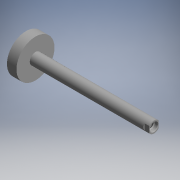
# Autodesk Inventor part: 536288 ADN-100-P-I_(KS)
Saved by Autodesk Inventor 2017.3 (Build 213256000, 256)
## iProperties
Part Number: 536288 ADN-100-P-I_(KS)
Material: Generic
Catalog Web Link: www.cadenas.de
Description: ADN-(KS)-Compact cylinder - piston rod
Vendor: FESTO
Document SubType Name: Modeling
Designer: partserver
Manufacturer: FESTO
Mass: 25.8333 g
Surface Area: 88.9082 cm^2
Volume: 25.8333 cm^3
Density: 1 g/cm^3
Appearance: PSOLRGB-191-191-191
Category: PARTsolutions
Company: FESTO
Title: 536288 ADN-100-P-I_(KS)
Author: Cadenas PARTsolutions
Comments: Compact cylinder - piston rod
PSOL_IDENT_0: {$CADENAS_DATA\23d-libs\festo\parts\a\adn\parts\adn_ks.prj},238 {VTYP=3D},{NB=536288 ADN-100-P-I_(KS
PSOL_IDENT_1: )},{LINA=536288 ADN-100-P-I_(KS)},{NN=ADN-(KS)},{DATE=20.11.2019 12:35:12},{GEOMDATE=08.01.2019 14:3
PSOL_IDENT_2: 4:57},{VERSION=},{LINEID=8210},{WBVAR=DF,HUB,TH,Q,S2S20,K2,K5,K8,K10,S1,TT,R8},{WBNUMERIC=HUB,K2,K8}
PSOL_IDENT_3: {NB=536288 ADN-100-P-I_(KS)},{LINA=536288 ADN-100-P-I_(KS)},{KT=536288},{TNR=536288},{AUSF=ADN},{D
PSOL_IDENT_4: F=P},{GA=A},{WHX=6.1},{WH0=6.100},{WH1=18.000},{WH2=12.500},{WH3=6.600},{WHX1=6.1},{WHX2=6.8},{WH=6.
PSOL_IDENT_5: 1},{ZM=58.600},{ZM2=59.700},{ZB=51.100},{ZB1=62.900},{ZB2=51.700},{ZB6=57.500},{ZA=45.000},{KDM=40},
PSOL_IDENT_6: {HUBP=-},{HUB=100},{HUB1=[1-400]},{HUB2=[1-300]},{HUB3=[10-400]},{HUB4=[1-400]},{TH=I},{THC='A','I'}
PSOL_IDENT_7: ,{Q=-},{VAR1C='-','Q'},{S2S20=-},{VAR2C='-','S2','S20'},{VAR22C='-','S2'},{VAR222C='-','S2'},{K2=0},
PSOL_IDENT_8: {VAR3C=0,[1-20]},{VAR33C=0},{K5=-},{K5A='-','M10','M12'},{K5I='-','M6'},{K5S1A='-','M10X1,25','M12'}
PSOL_IDENT_9: ,{K5S1I='-','M8'},{K5C='-','M6'},{K5N=0},{K5P=0},{K5T=},{K8=0},{K10=-},{K10A='-','K10'},{K10N=},{S1=
PSOL_IDENT_10: -},{TT=-},{TT1='-','TT'},{R8=-},{R81='-','R8'},{VAR4C=0,[1-400]},{VAR5C='-','S6'},{VAR6C='-','S1'},{
PSOL_IDENT_11: VAR66C='-','S1'},{VAR7C='-','R3'},{HUBALG=[1-400]},{A=19.000},{A1=22.000},{AF=16.000},{AF1=0.000},{A
PSOL_IDENT_12: F2=14.000},{AF3=20.000},{AF5=14.000},{AF7=16.000},{D8=4.500},{D9=8.000},{KF=M8},{KFN=8.000},{KF1=M10
PSOL_IDENT_13: },{KF1C=10.0000},{KF2=-},{KF2C=0.0000},{KF3=M6},{KF3C=6.0000},{KF5=M6},{KF5N=6},{KF7=M8},{KF7N=8},{K
PSOL_IDENT_14: K=M10X1.25},{KKN=10},{KKP=1.25},{KK1=M12X1.25},{KK1N=12.0000},{KK1P=1.25},{L2=45.000},{L8=3.000},{MM=
PSOL_IDENT_15: 12.000},{MM1=16.000},{PL=8.200},{SF=10},{SF1=13},{SF3=10.0},{WL=4.700},{WL1=6.500},{QN=},{S2N=},{S1N=
PSOL_IDENT_16: },{K2N=},{K8N=},{KKC3=8.200},{KKF2=0.600},{KKD5=1.500},{KKE2=20.000},{K5C3=0},{K5F2=0},{K5D5=0},{KK1
PSOL_IDENT_17: C3=10.200},{KK1F2=0.600},{KK1D5=1.500},{KK1E2=20.000},{L100S1=1.000},{L101S1=4.700},{L102S1=20.000},
PSOL_IDENT_18: {L103S1=24.000},{D100S1=10.500},{L100=0.400},{L101=3.300},{L102=16.000},{L103=20.000},{D100=8.400},{
PSOL_IDENT_19: L100Q=0.400},{L101Q=2.600},{L101K5=2.600},{L102Q=14.000},{L103Q=18.000},{D100Q=6.400},{L100S1K5=0.60
PSOL_IDENT_20: 0},{L101S1K5=3.300},{L102S1K5=16.000},{L103S1K5=21.000},{D100S1K5=8.400},{VERS=2},{TTN=},{R8N=},{D20=
PSOL_IDENT_21: 0.000},{XF31=4.000},{B31=5.000},{DFALG='P','PPS'}
NB: 536288 ADN-100-P-I_(KS)
NN: ADN-(KS)
NT: Compact cylinder - piston rod
NBSYN: $TNR. $AUSF.-$HUB.-$DF.-$TH.$QN.$S2N.$K2N.$K5T.$K8N.$K10N.$S1N.$TTN.$R8N._(KS)
LINA: 536288 ADN-100-P-I_(KS)
CATALOG: Festo
TNR: 536288
AUSF: ADN
DF: P
GA: A
WHX: 6.1
WH0: 6.1
WH1: 18
WH2: 12.5
WH3: 6.6
WHX1: 6.1
WHX2: 6.8
WH: 6.1
ZM: 58.6
ZM2: 59.7
ZB: 51.1
ZB1: 62.9
ZB2: 51.7
ZB6: 57.5
ZA: 45
KDM: 40
HUBP: -
HUB: 100
TH: I
Q: -
S2S20: -
K2: 0
K5: -
K8: 0
K10: -
S1: -
TT: -
R8: -
A: 19
A1: 22
AF: 16
AF1: 0
AF2: 14
AF3: 20
AF5: 14
AF7: 16
D8: 4.5
D9: 8
KF: M8
KF1: M10
KF2: -
KF3: M6
KF5: M6
KF7: M8
KK: M10X1.25
KK1: M12X1.25
L2: 45
L8: 3
MM: 12
MM1: 16
PL: 8.2
SF: 10
SF1: 13
SF3: 10
WL: 4.7
WL1: 6.5
L101K5: 2.6
D20: 0
XF31: 4
B31: 5
SUPPLIER: FESTO
ARTICLENO: 536288 ADN-100-P-I_(KS)
BOMINFO: 536288 ADN-100-P-I_(KS)
CREATOR: CADENAS GmbH
Autodesk Inventor part; units mm, degrees
sketch "Sketch_1" plane through (0, 0, 0) normal (0, 0, 1) x (1, 0, 0)
  line L0 (128.6, 0) -> (-6.1, 0)
  line L1 (-6.1, 0) -> (-6.1, 6)
  line L2 (-6.1, 6) -> (128.6, 6)
  line L3 (128.6, 6) -> (128.6, 0)
  line L4 (128.6, 0) -> (-6.1, 0)
  constraints: 10 end point
revolve "Revolution1" add sketch "Sketch_1" angle 360 about axis through (128.6, 0, 0) along (1, 0, 0)
sketch "Sketch_11" plane through (0, 0, 0) normal (0, 0, 1) x (1, 0, 0)
  line L0 (128.6, 0) -> (118.6, 0)
  line L1 (118.6, 0) -> (118.6, 20)
  line L2 (118.6, 20) -> (128.6, 20)
  line L3 (128.6, 20) -> (128.6, 0)
  line L4 (128.6, 0) -> (118.6, 0)
  constraints: 10 end point
revolve "Revolution2" add sketch "Sketch_11" angle 360 about axis through (128.6, 0, 0) along (1, 0, 0)
sketch "Sketch_20" plane through (0, 0, 0) normal (0, 0, 1) x (1, 0, 0)
  line L0 (-36.2, -16) -> (4.9509, -16)
  line L1 (4.9509, -16) -> (-1.4, -5)
  line L2 (-1.4, -5) -> (-6.1, -5)
  line L3 (-6.1, -5) -> (-6.1, -10)
  line L4 (-6.1, -10) -> (-30.1, -10)
  line L5 (-30.1, -10) -> (-30.1, 10)
  line L6 (-30.1, 10) -> (-6.1, 10)
  line L7 (-6.1, 10) -> (-6.1, 5)
  line L8 (-6.1, 5) -> (-1.4, 5)
  line L9 (-1.4, 5) -> (4.9509, 16)
  line L10 (4.9509, 16) -> (-36.2, 16)
  line L11 (-36.2, 16) -> (-36.2, -16)
  constraints: 24 end point
extrude "Extrusion1" cut sketch "Sketch_20" along normal mid plane 24
sketch "Sketch_2" plane through (0, 0, 0) normal (0, 0, 1) x (1, 0, 0)
  line L0 (15.8188, 0) -> (-6.1, 0)
  line L1 (-6.1, 0) -> (-6.1, 4.6)
  line L2 (-6.1, 4.6) -> (-5.7, 4.2)
  line L3 (-5.7, 4.2) -> (-2.8, 4.2)
  line L4 (-2.8, 4.2) -> (-2.8, 4)
  line L5 (-2.8, 4) -> (-2.1235, 3.3235)
  line L6 (-2.1235, 3.3235) -> (13.9, 3.3235)
  line L7 (13.9, 3.3235) -> (15.8188, 0)
  line L8 (15.8188, 0) -> (-6.1, 0)
  constraints: 18 end point
revolve "Revolution3" cut sketch "Sketch_2" angle 360 about axis through (15.8188, 0, 0) along (1, 0, 0)
thread "Thread1" size "M8x1.25" class "6H" standard "ISO Metric profile" length 12.0235
ref_plane "FDT_PIRODACC_F1_XY" through (-6.1, 0, 0) normal (-1, 0, 0) x (0, 1, 0)
ref_plane "FDT_PIRODACC_F1_YZ" through (-6.1, 0, 0) normal (0, 1, 0) x (0, 0, -1)
ref_plane "FDT_PIRODACC_F1_ZX" through (-6.1, 0, 0) normal (0, 0, -1) x (-1, 0, 0)
ref_plane "NUT1_XY" through (-12.6, 0, 0) normal (1, 0, 0) x (0, 0, -1)
ref_plane "NUT1_YZ" through (-12.6, 0, 0) normal (0, 0, -1) x (0, 1, 0)
ref_plane "NUT1_ZX" through (-12.6, 0, 0) normal (0, 1, 0) x (1, 0, 0)
ref_plane "PISTON_XY" through (128.6, 0, 0) normal (1, 0, 0) x (0, 0, -1)
ref_plane "PISTON_YZ" through (128.6, 0, 0) normal (0, 0, -1) x (0, 1, 0)
ref_plane "PISTON_ZX" through (128.6, 0, 0) normal (0, 1, 0) x (1, 0, 0)
body "Solid1"
